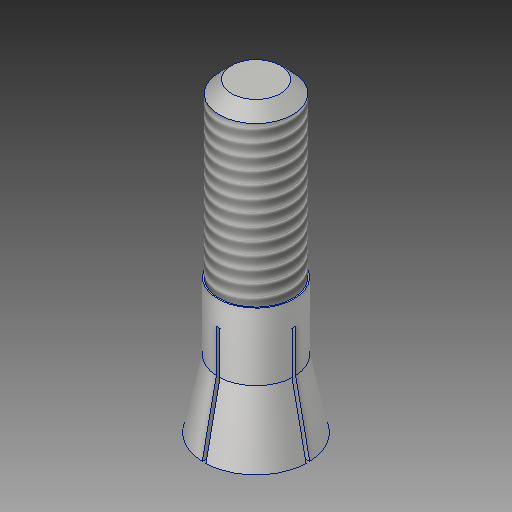
# Autodesk Inventor part: collet_screw
Saved by Autodesk Inventor 2018 (Build 220112000, 112)
## iProperties
Created: 2017-12-10
Part Number: collet_screw
Material: Aluminum 6061
Document SubType Name: Modeling
Designer: steve
Density: 2.7 g/cm^3
Appearance: Aluminum - Flat
Mass: 1.70054 g
Surface Area: 7.97215 cm^2
Volume: 0.629829 cm^3
Author: steve
Autodesk Inventor part; units mm, degrees
ref_plane "YZ Plane" through (0, 0, 0) normal (1, 0, 0) x (0, 1, 0)
ref_plane "XZ Plane" through (0, 0, 0) normal (0, 1, 0) x (-1, 0, 0)
ref_plane "XY Plane" through (0, 0, 0) normal (0, 0, 1) x (1, 0, 0)
sketch "Sketch1" plane through (0, 0, 0) normal (0, 0, 1) x (1, 0, 0)
  line L0 (0, 0) -> (-4.25, 0) construction
  line L1 (-4.25, 0) -> (-4.25, 5.5) construction
  line L2 (-4.25, 5.5) -> (0, 5.5) construction
  line L3 (0, 5.5) -> (0, 0) construction
  line L4 (0, 5.5) -> (-3.1, 5.5) construction
  line L5 (-3.1, 5.5) -> (-3.1, 11) construction
  line L6 (-3.1, 11) -> (0, 11) construction
  line L7 (0, 11) -> (0, 5.5) construction
  line L8 (0, 0) -> (-4.25, 0)
  line L9 (-4.25, 0) -> (-3.1, 5.5)
  line L10 (-3.1, 5.5) -> (-3.1, 11)
  line L11 (-3.1, 11) -> (0, 11)
  line L12 (0, 11) -> (0, 0)
  dimension "d0" = 5.5
  dimension "d1" = 4.25
  dimension "d2" = 5.5
  dimension "d3" = 3.1
  constraints: 26 end point, 4 parallel, 3 collinear, 3 horizontal, 2 perpendicular
  measures "d0" distance of L0.end L1.end
  measures "d1" distance of L1.end L2.end
  measures "d2" distance of L4.end L5.end
  measures "d3" distance of L5.end L6.end
revolve "Revolution1" add sketch "Sketch1" angle 360 about axis through (0, 11, 0) along (0, -1, 0)
sketch "Sketch2" plane through (0, 11, 0) normal (0, 1, 0) x (1, 0, 0)
  circle A0 centre (0, 0) radius 3
  circle A1 centre (0, 0) radius 3.1 construction
  dimension "d5" = 6
  constraints: 1 centre point, 1 coincident, 1 concentric
  measures "d5" diameter of A0
extrude "Extrusion1" add sketch "Sketch2" along normal blind 14
thread "Thread1" size "M6x1" class "6g" standard "ANSI Metric M Profile" full length
chamfer "Chamfer1" distance 1 angle 45 1 edges at (-3, 25, 0)
sketch "Sketch3" plane through (0, 0, 0) normal (0, -1, 0) x (1, 0, 0)
  point P0 (0, 0)
  point P1 (0, 0)
  constraints: 1 coincident
hole "Hole1" at (0, 0, 0) direction (0, 1, 0) diameter 4 depth 11 tip angle 118
sketch "Sketch4" plane through (0, 0, 0) normal (1, 0, 0) x (0, 1, 0)
  line L0 (0, -4.25) -> (0, 4.25) projected
  line L1 (0, 4.25) -> (9, 4.25)
  line L2 (9, 4.25) -> (9, -4.25)
  line L3 (9, -4.25) -> (0, -4.25)
  line L4 (0, -4.25) -> (0, 4.25)
  point P0 (0, 0)
  dimension "d20" = 9
  constraints: 8 end point, 2 parallel, 1 horizontal, 1 perpendicular, 1 point on line
  measures "d20" distance of L0.end L1.end
extrude "Extrusion2" cut sketch "Sketch4" along normal mid plane 0.3
sketch "Sketch5" plane through (0, 0, 0) normal (0, 0, 1) x (1, 0, 0)
  line L0 (4.25, 0) -> (3.1, 5.5) projected
  line L1 (4.25, 0) -> (-4.25, 0)
  line L2 (-4.25, 0) -> (-4.25, 9)
  line L3 (-4.25, 9) -> (4.25, 9)
  line L4 (4.25, 9) -> (4.25, 0)
  line L5 (0.15, 0) -> (0.15, 5.5) construction
  line L6 (0.15, 5.5) -> (0.15, 5.5) construction
  line L7 (0.15, 5.5) -> (0.15, 0) construction
  line L8 (0.15, 0) -> (0.15, 0) construction
  line L9 (-0.15, 5.5) -> (-0.15, 0) construction
  line L10 (-0.15, 0) -> (-0.15, 0) construction
  line L11 (-0.15, 0) -> (-0.15, 5.5) construction
  line L12 (-0.15, 5.5) -> (-0.15, 5.5) construction
  line L13 (-4.25, 0) -> (-3.1, 5.5) construction
  line L14 (-0.15, 0) -> (-4.25, 0) construction
  point P0 (0, 0)
  dimension "d23" = 9
  constraints: 8 end point, 3 point on line, 2 coincident, 2 parallel, 1 horizontal, 1 perpendicular
  measures "d23" distance of L1.end L2.end
extrude "Extrusion3" cut sketch "Sketch5" along normal mid plane 0.3
body "Solid1"
